Autodesk Inventor part; units mm, degrees
(part 2 of 2)
sketch "Sketch3" plane through (-0.0003, -144.9621, -142.4319) normal (0, 0, -1) x (-1, 0, 0)
  line L0 (-10.1604, 66.049) -> (-10.1604, 136.1421) construction
  line L1 (-10.1604, 136.1421) -> (-1.0068, 136.1421) construction
  line L2 (-1.0068, 136.1421) -> (-1.0068, 66.049) construction
  line L3 (-1.0068, 66.049) -> (-10.1604, 66.049) construction
  spline S0 degree 2 poles (-7.5802, 71.9161) (-7.0615, 71.9161) (-6.128, 71.5465) (-5.8038, 71.2159) knots 0 0 0 1 2 2 2
  spline S1 degree 2 poles (-5.8038, 71.2159) (-5.3954, 70.801) (-4.974, 69.6794) (-4.974, 68.8237) knots 0 0 0 1 2 2 2
  line L4 (-4.974, 68.8237) -> (-4.974, 67.9225)
  line L5 (-4.974, 67.9225) -> (-1.9918, 67.9225)
  line L6 (-1.9918, 67.9225) -> (-1.9918, 66.8593)
  line L7 (-1.9918, 66.8593) -> (-9.9918, 66.8593)
  line L8 (-9.9918, 66.8593) -> (-9.9918, 68.8691)
  spline S2 degree 2 poles (-9.9918, 68.8691) (-9.9918, 69.5822) (-9.7585, 70.5806) (-9.4927, 70.9631) knots 0 0 0 1 2 2 2
  spline S3 degree 2 poles (-9.4927, 70.9631) (-9.188, 71.4104) (-8.2479, 71.9161) (-7.5802, 71.9161) knots 0 0 0 1 2 2 2
  spline S4 degree 2 poles (-7.5478, 70.8075) (-7.9627, 70.8075) (-8.5721, 70.5222) (-8.7666, 70.2305) knots 0 0 0 1 2 2 2
  spline S5 degree 2 poles (-8.7666, 70.2305) (-8.9351, 69.9777) (-9.0713, 69.3034) (-9.0713, 68.8042) knots 0 0 0 1 2 2 2
  line L9 (-9.0713, 68.8042) -> (-9.0713, 67.9225)
  line L10 (-9.0713, 67.9225) -> (-5.8816, 67.9225)
  line L11 (-5.8816, 67.9225) -> (-5.8816, 68.6486)
  spline S6 degree 2 poles (-5.8816, 68.6486) (-5.8816, 69.2969) (-6.0891, 70.0943) (-6.3614, 70.3537) knots 0 0 0 1 2 2 2
  spline S7 degree 2 poles (-6.3614, 70.3537) (-6.6012, 70.5935) (-7.1653, 70.8075) (-7.5478, 70.8075) knots 0 0 0 1 2 2 2
  line L12 (-1.9918, 79.1187) -> (-1.9918, 77.7378)
  line L13 (-1.9918, 77.7378) -> (-5.175, 75.2094)
  line L14 (-5.175, 75.2094) -> (-5.175, 73.9906)
  line L15 (-5.175, 73.9906) -> (-1.9918, 73.9906)
  line L16 (-1.9918, 73.9906) -> (-1.9918, 72.9274)
  line L17 (-1.9918, 72.9274) -> (-9.9918, 72.9274)
  line L18 (-9.9918, 72.9274) -> (-9.9918, 74.989)
  spline S8 degree 2 poles (-9.9918, 74.989) (-9.9918, 75.6762) (-9.8427, 76.6033) (-9.5705, 77.0247) knots 0 0 0 1 2 2 2
  spline S9 degree 2 poles (-9.5705, 77.0247) (-9.2982, 77.446) (-8.4489, 77.9323) (-7.82, 77.9323) knots 0 0 0 1 2 2 2
  spline S10 degree 2 poles (-7.82, 77.9323) (-6.9448, 77.9323) (-5.7585, 77.0376) (-5.4732, 76.2726) knots 0 0 0 1 2 2 2
  line L19 (-5.4732, 76.2726) -> (-1.9918, 79.1187)
  spline S11 degree 2 poles (-7.7358, 76.8237) (-8.0858, 76.8237) (-8.6239, 76.5773) (-8.799, 76.318) knots 0 0 0 1 2 2 2
  spline S12 degree 2 poles (-8.799, 76.318) (-8.9481, 76.0911) (-9.0713, 75.4882) (-9.0713, 75.0473) knots 0 0 0 1 2 2 2
  line L20 (-9.0713, 75.0473) -> (-9.0713, 73.9906)
  line L21 (-9.0713, 73.9906) -> (-6.0632, 73.9906)
  line L22 (-6.0632, 73.9906) -> (-6.0632, 74.9242)
  spline S13 degree 2 poles (-6.0632, 74.9242) (-6.0632, 75.3845) (-6.2252, 76.117) (-6.4781, 76.3699) knots 0 0 0 1 2 2 2
  spline S14 degree 2 poles (-6.4781, 76.3699) (-6.6985, 76.6033) (-7.3209, 76.8237) (-7.7358, 76.8237) knots 0 0 0 1 2 2 2
  spline S15 degree 2 poles (-9.0777, 85.4136) (-8.5461, 85.8674) (-6.9902, 86.3731) (-5.9918, 86.3731) knots 0 0 0 1 2 2 2
  spline S16 degree 2 poles (-5.9918, 86.3731) (-5.0194, 86.3731) (-3.444, 85.8804) (-2.9124, 85.4136) knots 0 0 0 1 2 2 2
  spline S17 degree 2 poles (-2.9124, 85.4136) (-2.3549, 84.9209) (-1.8233, 83.6178) (-1.8233, 82.8334) knots 0 0 0 1 2 2 2
  spline S18 degree 2 poles (-1.8233, 82.8334) (-1.8233, 82.023) (-2.3743, 80.7264) (-2.9124, 80.2532) knots 0 0 0 1 2 2 2
  spline S19 degree 2 poles (-2.9124, 80.2532) (-3.444, 79.7929) (-5.0064, 79.3002) (-5.9918, 79.3002) knots 0 0 0 1 2 2 2
  spline S20 degree 2 poles (-5.9918, 79.3002) (-6.9967, 79.3002) (-8.5267, 79.7994) (-9.0777, 80.2597) knots 0 0 0 1 2 2 2
  spline S21 degree 2 poles (-9.0777, 80.2597) (-9.6094, 80.7264) (-10.1604, 82.0295) (-10.1604, 82.8334) knots 0 0 0 1 2 2 2
  spline S22 degree 2 poles (-10.1604, 82.8334) (-10.1604, 83.6503) (-9.5899, 84.9598) (-9.0777, 85.4136) knots 0 0 0 1 2 2 2
  spline S23 degree 2 poles (-5.9918, 85.2645) (-6.7828, 85.2645) (-8.0081, 84.9209) (-8.41, 84.6097) knots 0 0 0 1 2 2 2
  spline S24 degree 2 poles (-8.41, 84.6097) (-8.8249, 84.2921) (-9.2398, 83.3974) (-9.2398, 82.8399) knots 0 0 0 1 2 2 2
  spline S25 degree 2 poles (-9.2398, 82.8399) (-9.2398, 82.2629) (-8.8379, 81.3942) (-8.41, 81.0636) knots 0 0 0 1 2 2 2
  spline S26 degree 2 poles (-8.41, 81.0636) (-8.0016, 80.7459) (-6.7698, 80.4088) (-5.9918, 80.4088) knots 0 0 0 1 2 2 2
  spline S27 degree 2 poles (-5.9918, 80.4088) (-4.4165, 80.4088) (-2.7439, 81.7313) (-2.7439, 82.8399) knots 0 0 0 1 2 2 2
  spline S28 degree 2 poles (-2.7439, 82.8399) (-2.7439, 83.9485) (-4.4165, 85.2645) (-5.9918, 85.2645) knots 0 0 0 1 2 2 2
  line L23 (-1.9918, 89.4071) -> (-9.0453, 89.4071)
  line L24 (-9.0453, 89.4071) -> (-9.0453, 86.7232)
  line L25 (-9.0453, 86.7232) -> (-9.9918, 86.7232)
  line L26 (-9.9918, 86.7232) -> (-9.9918, 93.1543)
  line L27 (-9.9918, 93.1543) -> (-9.0453, 93.1543)
  line L28 (-9.0453, 93.1543) -> (-9.0453, 90.4704)
  line L29 (-9.0453, 90.4704) -> (-1.9918, 90.4704)
  line L30 (-1.9918, 90.4704) -> (-1.9918, 89.4071)
  spline S29 degree 2 poles (-9.0777, 99.6243) (-8.5461, 100.0781) (-6.9902, 100.5838) (-5.9918, 100.5838) knots 0 0 0 1 2 2 2
  spline S30 degree 2 poles (-5.9918, 100.5838) (-5.0194, 100.5838) (-3.444, 100.0911) (-2.9124, 99.6243) knots 0 0 0 1 2 2 2
  spline S31 degree 2 poles (-2.9124, 99.6243) (-2.3549, 99.1316) (-1.8233, 97.8285) (-1.8233, 97.0441) knots 0 0 0 1 2 2 2
  spline S32 degree 2 poles (-1.8233, 97.0441) (-1.8233, 96.2337) (-2.3743, 94.9371) (-2.9124, 94.4639) knots 0 0 0 1 2 2 2
  spline S33 degree 2 poles (-2.9124, 94.4639) (-3.444, 94.0036) (-5.0064, 93.5109) (-5.9918, 93.5109) knots 0 0 0 1 2 2 2
  spline S34 degree 2 poles (-5.9918, 93.5109) (-6.9967, 93.5109) (-8.5267, 94.0101) (-9.0777, 94.4704) knots 0 0 0 1 2 2 2
  spline S35 degree 2 poles (-9.0777, 94.4704) (-9.6094, 94.9371) (-10.1604, 96.2402) (-10.1604, 97.0441) knots 0 0 0 1 2 2 2
  spline S36 degree 2 poles (-10.1604, 97.0441) (-10.1604, 97.861) (-9.5899, 99.1705) (-9.0777, 99.6243) knots 0 0 0 1 2 2 2
  spline S37 degree 2 poles (-5.9918, 99.4752) (-6.7828, 99.4752) (-8.0081, 99.1316) (-8.41, 98.8204) knots 0 0 0 1 2 2 2
  spline S38 degree 2 poles (-8.41, 98.8204) (-8.8249, 98.5028) (-9.2398, 97.6081) (-9.2398, 97.0506) knots 0 0 0 1 2 2 2
  spline S39 degree 2 poles (-9.2398, 97.0506) (-9.2398, 96.4736) (-8.8379, 95.6049) (-8.41, 95.2742) knots 0 0 0 1 2 2 2
  spline S40 degree 2 poles (-8.41, 95.2742) (-8.0016, 94.9566) (-6.7698, 94.6195) (-5.9918, 94.6195) knots 0 0 0 1 2 2 2
  spline S41 degree 2 poles (-5.9918, 94.6195) (-4.4165, 94.6195) (-2.7439, 95.942) (-2.7439, 97.0506) knots 0 0 0 1 2 2 2
  spline S42 degree 2 poles (-2.7439, 97.0506) (-2.7439, 98.1592) (-4.4165, 99.4752) (-5.9918, 99.4752) knots 0 0 0 1 2 2 2
  line L31 (-1.9918, 103.6178) -> (-9.0453, 103.6178)
  line L32 (-9.0453, 103.6178) -> (-9.0453, 100.9339)
  line L33 (-9.0453, 100.9339) -> (-9.9918, 100.9339)
  line L34 (-9.9918, 100.9339) -> (-9.9918, 107.365)
  line L35 (-9.9918, 107.365) -> (-9.0453, 107.365)
  line L36 (-9.0453, 107.365) -> (-9.0453, 104.6811)
  line L37 (-9.0453, 104.6811) -> (-1.9918, 104.6811)
  line L38 (-1.9918, 104.6811) -> (-1.9918, 103.6178)
  line L39 (-9.9918, 113.7767) -> (-5.5316, 111.0733)
  line L40 (-5.5316, 111.0733) -> (-1.9918, 111.0733)
  line L41 (-1.9918, 111.0733) -> (-1.9918, 110.0101)
  line L42 (-1.9918, 110.0101) -> (-5.4213, 110.0101)
  line L43 (-5.4213, 110.0101) -> (-9.9918, 107.3067)
  line L44 (-9.9918, 107.3067) -> (-9.9918, 108.4866)
  line L45 (-9.9918, 108.4866) -> (-6.4716, 110.5482)
  line L46 (-6.4716, 110.5482) -> (-9.9918, 112.6486)
  line L47 (-9.9918, 112.6486) -> (-9.9918, 113.7767)
  spline S43 degree 2 poles (-7.5802, 119.5725) (-7.0615, 119.5725) (-6.128, 119.2029) (-5.8038, 118.8723) knots 0 0 0 1 2 2 2
  spline S44 degree 2 poles (-5.8038, 118.8723) (-5.3954, 118.4574) (-4.974, 117.3358) (-4.974, 116.4801) knots 0 0 0 1 2 2 2
  line L48 (-4.974, 116.4801) -> (-4.974, 115.5789)
  line L49 (-4.974, 115.5789) -> (-1.9918, 115.5789)
  line L50 (-1.9918, 115.5789) -> (-1.9918, 114.5157)
  line L51 (-1.9918, 114.5157) -> (-9.9918, 114.5157)
  line L52 (-9.9918, 114.5157) -> (-9.9918, 116.5255)
  spline S45 degree 2 poles (-9.9918, 116.5255) (-9.9918, 117.2386) (-9.7585, 118.237) (-9.4927, 118.6195) knots 0 0 0 1 2 2 2
  spline S46 degree 2 poles (-9.4927, 118.6195) (-9.188, 119.0668) (-8.2479, 119.5725) (-7.5802, 119.5725) knots 0 0 0 1 2 2 2
  spline S47 degree 2 poles (-7.5478, 118.4639) (-7.9627, 118.4639) (-8.5721, 118.1786) (-8.7666, 117.8869) knots 0 0 0 1 2 2 2
  spline S48 degree 2 poles (-8.7666, 117.8869) (-8.9351, 117.6341) (-9.0713, 116.9598) (-9.0713, 116.4606) knots 0 0 0 1 2 2 2
  line L53 (-9.0713, 116.4606) -> (-9.0713, 115.5789)
  line L54 (-9.0713, 115.5789) -> (-5.8816, 115.5789)
  line L55 (-5.8816, 115.5789) -> (-5.8816, 116.305)
  spline S49 degree 2 poles (-5.8816, 116.305) (-5.8816, 116.9533) (-6.0891, 117.7507) (-6.3614, 118.0101) knots 0 0 0 1 2 2 2
  spline S50 degree 2 poles (-6.3614, 118.0101) (-6.6012, 118.2499) (-7.1653, 118.4639) (-7.5478, 118.4639) knots 0 0 0 1 2 2 2
  line L56 (-1.9918, 120.5838) -> (-9.9918, 120.5838)
  line L57 (-9.9918, 120.5838) -> (-9.9918, 125.5887)
  line L58 (-9.9918, 125.5887) -> (-9.0453, 125.5887)
  line L59 (-9.0453, 125.5887) -> (-9.0453, 121.647)
  line L60 (-9.0453, 121.647) -> (-6.8541, 121.647)
  line L61 (-6.8541, 121.647) -> (-6.8541, 125.3229)
  line L62 (-6.8541, 125.3229) -> (-5.9076, 125.3229)
  line L63 (-5.9076, 125.3229) -> (-5.9076, 121.647)
  line L64 (-5.9076, 121.647) -> (-2.9384, 121.647)
  line L65 (-2.9384, 121.647) -> (-2.9384, 125.5887)
  line L66 (-2.9384, 125.5887) -> (-1.9918, 125.5887)
  line L67 (-1.9918, 125.5887) -> (-1.9918, 120.5838)
  spline S51 degree 2 poles (-4.5332, 134.814) (-3.9562, 134.814) (-2.9708, 134.4444) (-2.6077, 134.1073) knots 0 0 0 1 2 2 2
  spline S52 degree 2 poles (-2.6077, 134.1073) (-2.2447, 133.7702) (-1.8233, 132.7653) (-1.8233, 132.143) knots 0 0 0 1 2 2 2
  spline S53 degree 2 poles (-1.8233, 132.143) (-1.8233, 131.5725) (-2.0761, 130.4574) (-2.2771, 130.049) knots 0 0 0 1 2 2 2
  line L68 (-2.2771, 130.049) -> (-3.4116, 130.049)
  line L69 (-3.4116, 130.049) -> (-3.4116, 130.1268)
  spline S54 degree 2 poles (-3.4116, 130.1268) (-3.3209, 130.2499) (-3.0875, 130.7102) (-2.9837, 130.989) knots 0 0 0 1 2 2 2
  spline S55 degree 2 poles (-2.9837, 130.989) (-2.8735, 131.3067) (-2.7504, 131.8318) (-2.7504, 132.1624) knots 0 0 0 1 2 2 2
  spline S56 degree 2 poles (-2.7504, 132.1624) (-2.7504, 132.4866) (-2.9837, 133.096) (-3.2366, 133.3164) knots 0 0 0 1 2 2 2
  spline S57 degree 2 poles (-3.2366, 133.3164) (-3.4764, 133.5174) (-4.1118, 133.7248) (-4.5397, 133.7248) knots 0 0 0 1 2 2 2
  spline S58 degree 2 poles (-4.5397, 133.7248) (-4.9675, 133.7248) (-5.5121, 133.4914) (-5.6936, 133.271) knots 0 0 0 1 2 2 2
  spline S59 degree 2 poles (-5.6936, 133.271) (-5.8946, 133.0441) (-6.0632, 132.3699) (-6.0632, 131.9614) knots 0 0 0 1 2 2 2
  spline S60 degree 2 poles (-6.0632, 131.9614) (-6.0632, 131.5206) (-5.927, 130.6454) (-5.8687, 130.3796) knots 0 0 0 1 2 2 2
  line L70 (-5.8687, 130.3796) -> (-9.9918, 130.3796)
  line L71 (-9.9918, 130.3796) -> (-9.9918, 134.7686)
  line L72 (-9.9918, 134.7686) -> (-9.0518, 134.7686)
  line L73 (-9.0518, 134.7686) -> (-9.0518, 131.4104)
  line L74 (-9.0518, 131.4104) -> (-6.9189, 131.4104)
  spline S61 degree 2 poles (-6.9189, 131.4104) (-6.9448, 131.6049) (-6.9643, 131.9809) (-6.9643, 132.1365) knots 0 0 0 1 2 2 2
  spline S62 degree 2 poles (-6.9643, 132.1365) (-6.9643, 132.7524) (-6.7633, 133.6016) (-6.4651, 133.9906) knots 0 0 0 1 2 2 2
  spline S63 degree 2 poles (-6.4651, 133.9906) (-6.1669, 134.3861) (-5.2593, 134.814) (-4.5332, 134.814) knots 0 0 0 1 2 2 2
  point P0 (-0.0003, 144.9621)
  constraints: 2 other
extrude "Extrusion3" add sketch "Sketch3" against normal blind 2
ref_plane "Work Plane4" through (-0.0003, -144.9621, 0) normal (-0.0000018, -1, 0) x (-0.0015858, 0, -0.9999987)
sketch "Sketch4" plane through (-0.0003, -144.9621, 0) normal (-0.0000018, -1, 0) x (-0.0015858, 0, -0.9999987)
  line L0 (16.9376, 64.7399) -> (58.7136, 64.7399) construction
  line L1 (58.7136, 64.7399) -> (58.7136, 48.1903) construction
  line L2 (58.7136, 48.1903) -> (16.9376, 48.1903) construction
  line L3 (16.9376, 48.1903) -> (16.9376, 64.7399) construction
  line L4 (19.529, 58.6329) -> (17.2049, 58.6329)
  line L5 (17.2049, 58.6329) -> (17.2049, 59.2456)
  line L6 (17.2049, 59.2456) -> (17.9682, 59.2456)
  line L7 (17.9682, 59.2456) -> (17.9682, 64.0203)
  line L8 (17.9682, 64.0203) -> (17.2049, 64.0203)
  line L9 (17.2049, 64.0203) -> (17.2049, 64.6329)
  line L10 (17.2049, 64.6329) -> (19.529, 64.6329)
  line L11 (19.529, 64.6329) -> (19.529, 64.0203)
  line L12 (19.529, 64.0203) -> (18.7656, 64.0203)
  line L13 (18.7656, 64.0203) -> (18.7656, 59.2456)
  line L14 (18.7656, 59.2456) -> (19.529, 59.2456)
  line L15 (19.529, 59.2456) -> (19.529, 58.6329)
  line L16 (24.8094, 58.6329) -> (23.9148, 58.6329)
  line L17 (23.9148, 58.6329) -> (21.26, 63.8063)
  line L18 (21.26, 63.8063) -> (21.26, 58.6329)
  line L19 (21.26, 58.6329) -> (20.5161, 58.6329)
  line L20 (20.5161, 58.6329) -> (20.5161, 64.6329)
  line L21 (20.5161, 64.6329) -> (21.649, 64.6329)
  line L22 (21.649, 64.6329) -> (24.0655, 59.8825)
  line L23 (24.0655, 59.8825) -> (24.0655, 64.6329)
  line L24 (24.0655, 64.6329) -> (24.8094, 64.6329)
  line L25 (24.8094, 64.6329) -> (24.8094, 58.6329)
  line L26 (27.4253, 58.6329) -> (27.4253, 63.923)
  line L27 (27.4253, 63.923) -> (25.4123, 63.923)
  line L28 (25.4123, 63.923) -> (25.4123, 64.6329)
  line L29 (25.4123, 64.6329) -> (30.2357, 64.6329)
  line L30 (30.2357, 64.6329) -> (30.2357, 63.923)
  line L31 (30.2357, 63.923) -> (28.2227, 63.923)
  line L32 (28.2227, 63.923) -> (28.2227, 58.6329)
  line L33 (28.2227, 58.6329) -> (27.4253, 58.6329)
  line L34 (30.8434, 58.6329) -> (30.8434, 64.6329)
  line L35 (30.8434, 64.6329) -> (34.5971, 64.6329)
  line L36 (34.5971, 64.6329) -> (34.5971, 63.923)
  line L37 (34.5971, 63.923) -> (31.6409, 63.923)
  line L38 (31.6409, 63.923) -> (31.6409, 62.2796)
  line L39 (31.6409, 62.2796) -> (34.3977, 62.2796)
  line L40 (34.3977, 62.2796) -> (34.3977, 61.5697)
  line L41 (34.3977, 61.5697) -> (31.6409, 61.5697)
  line L42 (31.6409, 61.5697) -> (31.6409, 59.3428)
  line L43 (31.6409, 59.3428) -> (34.5971, 59.3428)
  line L44 (34.5971, 59.3428) -> (34.5971, 58.6329)
  line L45 (34.5971, 58.6329) -> (30.8434, 58.6329)
  line L46 (40.1157, 58.6329) -> (39.0801, 58.6329)
  line L47 (39.0801, 58.6329) -> (37.1838, 61.0203)
  line L48 (37.1838, 61.0203) -> (36.2697, 61.0203)
  line L49 (36.2697, 61.0203) -> (36.2697, 58.6329)
  line L50 (36.2697, 58.6329) -> (35.4723, 58.6329)
  line L51 (35.4723, 58.6329) -> (35.4723, 64.6329)
  line L52 (35.4723, 64.6329) -> (37.0185, 64.6329)
  spline S0 degree 2 poles (37.0185, 64.6329) (37.5339, 64.6329) (38.2292, 64.5211) (38.5452, 64.3169) knots 0 0 0 1 2 2 2
  spline S1 degree 2 poles (38.5452, 64.3169) (38.8613, 64.1127) (39.2259, 63.4757) (39.2259, 63.0041) knots 0 0 0 1 2 2 2
  spline S2 degree 2 poles (39.2259, 63.0041) (39.2259, 62.3477) (38.555, 61.4579) (37.9812, 61.2439) knots 0 0 0 1 2 2 2
  line L53 (37.9812, 61.2439) -> (40.1157, 58.6329)
  spline S3 degree 2 poles (38.3945, 62.9409) (38.3945, 63.2034) (38.2097, 63.607) (38.0152, 63.7383) knots 0 0 0 1 2 2 2
  spline S4 degree 2 poles (38.0152, 63.7383) (37.8451, 63.8501) (37.3929, 63.9425) (37.0622, 63.9425) knots 0 0 0 1 2 2 2
  line L54 (37.0622, 63.9425) -> (36.2697, 63.9425)
  line L55 (36.2697, 63.9425) -> (36.2697, 61.6864)
  line L56 (36.2697, 61.6864) -> (36.9699, 61.6864)
  spline S5 degree 2 poles (36.9699, 61.6864) (37.3151, 61.6864) (37.8645, 61.808) (38.0541, 61.9976) knots 0 0 0 1 2 2 2
  spline S6 degree 2 poles (38.0541, 61.9976) (38.2292, 62.1629) (38.3945, 62.6297) (38.3945, 62.9409) knots 0 0 0 1 2 2 2
  line L57 (44.1806, 63.923) -> (41.3896, 63.923)
  line L58 (41.3896, 63.923) -> (41.3896, 62.231)
  line L59 (41.3896, 62.231) -> (44.0639, 62.231)
  line L60 (44.0639, 62.231) -> (44.0639, 61.5211)
  line L61 (44.0639, 61.5211) -> (41.3896, 61.5211)
  line L62 (41.3896, 61.5211) -> (41.3896, 58.6329)
  line L63 (41.3896, 58.6329) -> (40.5922, 58.6329)
  line L64 (40.5922, 58.6329) -> (40.5922, 64.6329)
  line L65 (40.5922, 64.6329) -> (44.1806, 64.6329)
  line L66 (44.1806, 64.6329) -> (44.1806, 63.923)
  line L67 (44.2486, 58.6329) -> (46.2713, 64.6329)
  line L68 (46.2713, 64.6329) -> (47.2535, 64.6329)
  line L69 (47.2535, 64.6329) -> (49.2762, 58.6329)
  line L70 (49.2762, 58.6329) -> (48.435, 58.6329)
  line L71 (48.435, 58.6329) -> (47.8904, 60.3104)
  line L72 (47.8904, 60.3104) -> (45.6003, 60.3104)
  line L73 (45.6003, 60.3104) -> (45.0558, 58.6329)
  line L74 (45.0558, 58.6329) -> (44.2486, 58.6329)
  line L75 (47.6716, 60.9911) -> (46.743, 63.8161)
  line L76 (46.743, 63.8161) -> (45.8191, 60.9911)
  line L77 (45.8191, 60.9911) -> (47.6716, 60.9911)
  spline S7 degree 2 poles (52.1887, 58.5259) (51.6052, 58.5259) (50.6182, 58.9198) (50.2584, 59.3136) knots 0 0 0 1 2 2 2
  spline S8 degree 2 poles (50.2584, 59.3136) (49.8986, 59.7026) (49.5047, 60.8695) (49.5047, 61.6281) knots 0 0 0 1 2 2 2
  spline S9 degree 2 poles (49.5047, 61.6281) (49.5047, 62.3817) (49.8888, 63.5) (50.2535, 63.9133) knots 0 0 0 1 2 2 2
  spline S10 degree 2 poles (50.2535, 63.9133) (50.6133, 64.3169) (51.5955, 64.7399) (52.2033, 64.7399) knots 0 0 0 1 2 2 2
  spline S11 degree 2 poles (52.2033, 64.7399) (52.5047, 64.7399) (53.0347, 64.6524) (53.2584, 64.5843) knots 0 0 0 1 2 2 2
  spline S12 degree 2 poles (53.2584, 64.5843) (53.4528, 64.5211) (53.8564, 64.3412) (54.0558, 64.2342) knots 0 0 0 1 2 2 2
  line L78 (54.0558, 64.2342) -> (54.0558, 63.2715)
  line L79 (54.0558, 63.2715) -> (53.9926, 63.2715)
  spline S13 degree 2 poles (53.9926, 63.2715) (53.8856, 63.3687) (53.555, 63.641) (53.3167, 63.7723) knots 0 0 0 1 2 2 2
  spline S14 degree 2 poles (53.3167, 63.7723) (53.0882, 63.8987) (52.5485, 64.0592) (52.1984, 64.0592) knots 0 0 0 1 2 2 2
  spline S15 degree 2 poles (52.1984, 64.0592) (51.8143, 64.0592) (51.1287, 63.7431) (50.871, 63.4417) knots 0 0 0 1 2 2 2
  spline S16 degree 2 poles (50.871, 63.4417) (50.6182, 63.1353) (50.3362, 62.2067) (50.3362, 61.6281) knots 0 0 0 1 2 2 2
  spline S17 degree 2 poles (50.3362, 61.6281) (50.3362, 61.0106) (50.6327, 60.1208) (50.8904, 59.8144) knots 0 0 0 1 2 2 2
  spline S18 degree 2 poles (50.8904, 59.8144) (51.1433, 59.5178) (51.8191, 59.2164) (52.1984, 59.2164) knots 0 0 0 1 2 2 2
  spline S19 degree 2 poles (52.1984, 59.2164) (52.5436, 59.2164) (53.1319, 59.3866) (53.3605, 59.513) knots 0 0 0 1 2 2 2
  spline S20 degree 2 poles (53.3605, 59.513) (53.5793, 59.6394) (53.905, 59.902) (53.9974, 59.9943) knots 0 0 0 1 2 2 2
  line L80 (53.9974, 59.9943) -> (54.0558, 59.9943)
  line L81 (54.0558, 59.9943) -> (54.0558, 59.0413)
  spline S21 degree 2 poles (54.0558, 59.0413) (53.8564, 58.949) (53.5063, 58.7788) (53.2584, 58.701) knots 0 0 0 1 2 2 2
  spline S22 degree 2 poles (53.2584, 58.701) (52.9958, 58.6135) (52.5485, 58.5259) (52.1887, 58.5259) knots 0 0 0 1 2 2 2
  line L82 (54.7997, 58.6329) -> (54.7997, 64.6329)
  line L83 (54.7997, 64.6329) -> (58.5533, 64.6329)
  line L84 (58.5533, 64.6329) -> (58.5533, 63.923)
  line L85 (58.5533, 63.923) -> (55.5971, 63.923)
  line L86 (55.5971, 63.923) -> (55.5971, 62.2796)
  line L87 (55.5971, 62.2796) -> (58.354, 62.2796)
  line L88 (58.354, 62.2796) -> (58.354, 61.5697)
  line L89 (58.354, 61.5697) -> (55.5971, 61.5697)
  line L90 (55.5971, 61.5697) -> (55.5971, 59.3428)
  line L91 (55.5971, 59.3428) -> (58.5533, 59.3428)
  line L92 (58.5533, 59.3428) -> (58.5533, 58.6329)
  line L93 (58.5533, 58.6329) -> (54.7997, 58.6329)
  line L94 (27.6076, 48.7541) -> (26.8102, 48.7541)
  line L95 (26.8102, 48.7541) -> (26.8102, 53.9226)
  line L96 (26.8102, 53.9226) -> (25.2446, 50.4072)
  line L97 (25.2446, 50.4072) -> (24.7584, 50.4072)
  line L98 (24.7584, 50.4072) -> (23.2073, 53.9226)
  line L99 (23.2073, 53.9226) -> (23.2073, 48.7541)
  line L100 (23.2073, 48.7541) -> (22.4634, 48.7541)
  line L101 (22.4634, 48.7541) -> (22.4634, 54.7541)
  line L102 (22.4634, 54.7541) -> (23.5525, 54.7541)
  line L103 (23.5525, 54.7541) -> (25.0501, 51.4137)
  line L104 (25.0501, 51.4137) -> (26.499, 54.7541)
  line L105 (26.499, 54.7541) -> (27.6076, 54.7541)
  line L106 (27.6076, 54.7541) -> (27.6076, 48.7541)
  spline S23 degree 2 poles (33.0679, 54.0685) (33.4083, 53.6698) (33.7875, 52.5029) (33.7875, 51.7541) knots 0 0 0 1 2 2 2
  spline S24 degree 2 poles (33.7875, 51.7541) (33.7875, 51.0247) (33.418, 49.8432) (33.0679, 49.4445) knots 0 0 0 1 2 2 2
  spline S25 degree 2 poles (33.0679, 49.4445) (32.6984, 49.0264) (31.7211, 48.6277) (31.1327, 48.6277) knots 0 0 0 1 2 2 2
  spline S26 degree 2 poles (31.1327, 48.6277) (30.525, 48.6277) (29.5525, 49.0409) (29.1976, 49.4445) knots 0 0 0 1 2 2 2
  spline S27 degree 2 poles (29.1976, 49.4445) (28.8524, 49.8432) (28.4828, 51.015) (28.4828, 51.7541) knots 0 0 0 1 2 2 2
  spline S28 degree 2 poles (28.4828, 51.7541) (28.4828, 52.5077) (28.8572, 53.6552) (29.2024, 54.0685) knots 0 0 0 1 2 2 2
  spline S29 degree 2 poles (29.2024, 54.0685) (29.5525, 54.4672) (30.5298, 54.8805) (31.1327, 54.8805) knots 0 0 0 1 2 2 2
  spline S30 degree 2 poles (31.1327, 54.8805) (31.7454, 54.8805) (32.7276, 54.4526) (33.0679, 54.0685) knots 0 0 0 1 2 2 2
  spline S31 degree 2 poles (32.9561, 51.7541) (32.9561, 52.3473) (32.6984, 53.2662) (32.465, 53.5677) knots 0 0 0 1 2 2 2
  spline S32 degree 2 poles (32.465, 53.5677) (32.2268, 53.8789) (31.5558, 54.1901) (31.1376, 54.1901) knots 0 0 0 1 2 2 2
  spline S33 degree 2 poles (31.1376, 54.1901) (30.7049, 54.1901) (30.0533, 53.8886) (29.8054, 53.5677) knots 0 0 0 1 2 2 2
  spline S34 degree 2 poles (29.8054, 53.5677) (29.5671, 53.2614) (29.3143, 52.3375) (29.3143, 51.7541) knots 0 0 0 1 2 2 2
  spline S35 degree 2 poles (29.3143, 51.7541) (29.3143, 50.5726) (30.3062, 49.3181) (31.1376, 49.3181) knots 0 0 0 1 2 2 2
  spline S36 degree 2 poles (31.1376, 49.3181) (31.9691, 49.3181) (32.9561, 50.5726) (32.9561, 51.7541) knots 0 0 0 1 2 2 2
  spline S37 degree 2 poles (39.3937, 51.7492) (39.3937, 50.9275) (38.7276, 49.605) (38.1684, 49.2354) knots 0 0 0 1 2 2 2
  spline S38 degree 2 poles (38.1684, 49.2354) (37.7114, 48.9486) (36.7729, 48.7541) (36.0436, 48.7541) knots 0 0 0 1 2 2 2
  line L107 (36.0436, 48.7541) -> (34.6627, 48.7541)
  line L108 (34.6627, 48.7541) -> (34.6627, 54.7541)
  line L109 (34.6627, 54.7541) -> (36.029, 54.7541)
  spline S39 degree 2 poles (36.029, 54.7541) (36.8751, 54.7541) (37.8378, 54.5012) (38.1781, 54.2776) knots 0 0 0 1 2 2 2
  spline S40 degree 2 poles (38.1781, 54.2776) (38.7567, 53.8935) (39.3937, 52.6244) (39.3937, 51.7492) knots 0 0 0 1 2 2 2
  spline S41 degree 2 poles (38.5622, 51.7589) (38.5622, 52.4494) (38.1052, 53.4267) (37.653, 53.7038) knots 0 0 0 1 2 2 2
  spline S42 degree 2 poles (37.653, 53.7038) (37.3321, 53.8935) (36.6076, 54.0636) (36.0679, 54.0636) knots 0 0 0 1 2 2 2
  line L110 (36.0679, 54.0636) -> (35.4601, 54.0636)
  line L111 (35.4601, 54.0636) -> (35.4601, 49.4445)
  line L112 (35.4601, 49.4445) -> (36.0679, 49.4445)
  spline S43 degree 2 poles (36.0679, 49.4445) (36.5979, 49.4445) (37.4002, 49.6147) (37.7259, 49.8432) knots 0 0 0 1 2 2 2
  spline S44 degree 2 poles (37.7259, 49.8432) (38.1441, 50.1252) (38.5622, 51.0588) (38.5622, 51.7589) knots 0 0 0 1 2 2 2
  spline S45 degree 2 poles (42.3548, 48.6277) (41.8248, 48.6277) (41.0371, 48.9048) (40.76, 49.182) knots 0 0 0 1 2 2 2
  spline S46 degree 2 poles (40.76, 49.182) (40.4439, 49.4931) (40.1862, 50.3683) (40.1862, 51.0102) knots 0 0 0 1 2 2 2
  line L113 (40.1862, 51.0102) -> (40.1862, 54.7541)
  line L114 (40.1862, 54.7541) -> (40.9836, 54.7541)
  line L115 (40.9836, 54.7541) -> (40.9836, 51.0102)
  spline S47 degree 2 poles (40.9836, 51.0102) (40.9836, 50.592) (41.0906, 50.028) (41.2413, 49.7995) knots 0 0 0 1 2 2 2
  spline S48 degree 2 poles (41.2413, 49.7995) (41.4018, 49.5563) (41.9561, 49.3084) (42.3548, 49.3084) knots 0 0 0 1 2 2 2
  spline S49 degree 2 poles (42.3548, 49.3084) (42.7292, 49.3084) (43.3127, 49.5563) (43.4731, 49.7995) knots 0 0 0 1 2 2 2
  spline S50 degree 2 poles (43.4731, 49.7995) (43.6238, 50.028) (43.7308, 50.5871) (43.7308, 50.9907) knots 0 0 0 1 2 2 2
  line L116 (43.7308, 50.9907) -> (43.7308, 54.7541)
  line L117 (43.7308, 54.7541) -> (44.5282, 54.7541)
  line L118 (44.5282, 54.7541) -> (44.5282, 51.0102)
  spline S51 degree 2 poles (44.5282, 51.0102) (44.5282, 50.3829) (44.2754, 49.4883) (43.9545, 49.182) knots 0 0 0 1 2 2 2
  spline S52 degree 2 poles (43.9545, 49.182) (43.6676, 48.8999) (42.9091, 48.6277) (42.3548, 48.6277) knots 0 0 0 1 2 2 2
  line L119 (49.1473, 48.7541) -> (45.6708, 48.7541)
  line L120 (45.6708, 48.7541) -> (45.6708, 54.7541)
  line L121 (45.6708, 54.7541) -> (46.4682, 54.7541)
  line L122 (46.4682, 54.7541) -> (46.4682, 49.464)
  line L123 (46.4682, 49.464) -> (49.1473, 49.464)
  line L124 (49.1473, 49.464) -> (49.1473, 48.7541)
  line L125 (49.7746, 48.7541) -> (49.7746, 54.7541)
  line L126 (49.7746, 54.7541) -> (53.5282, 54.7541)
  line L127 (53.5282, 54.7541) -> (53.5282, 54.0442)
  line L128 (53.5282, 54.0442) -> (50.572, 54.0442)
  line L129 (50.572, 54.0442) -> (50.572, 52.4008)
  line L130 (50.572, 52.4008) -> (53.3289, 52.4008)
  line L131 (53.3289, 52.4008) -> (53.3289, 51.6909)
  line L132 (53.3289, 51.6909) -> (50.572, 51.6909)
  line L133 (50.572, 51.6909) -> (50.572, 49.464)
  line L134 (50.572, 49.464) -> (53.5282, 49.464)
  line L135 (53.5282, 49.464) -> (53.5282, 48.7541)
  line L136 (53.5282, 48.7541) -> (49.7746, 48.7541)
  point P0 (0, 0)
  constraints: 2 other
extrude "Extrusion4" add sketch "Sketch4" against normal blind 2
body "Solid1"
